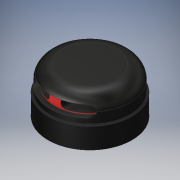
# Autodesk Inventor part: RPLidar A2
Saved by Autodesk Inventor 2018 (Build 220112000, 112)
## iProperties
Part Number: RPLidar A2
Material: Generisch
Document SubType Name: Modeling
Designer: Jochen Alt
Mass: 156.122 g
Surface Area: 240.31 cm^2
Volume: 156.122 cm^3
Density: 1 g/cm^3
Appearance: Glänzend - schwarz
Author: Jochen Alt
Autodesk Inventor part; units mm, degrees
ref_plane "YZ Plane" through (0, 0, 0) normal (1, 0, 0) x (0, 1, 0)
ref_plane "XZ Plane" through (0, 0, 0) normal (0, 1, 0) x (-1, 0, 0)
ref_plane "XY Plane" through (0, 0, 0) normal (0, 0, 1) x (1, 0, 0)
sketch "Skizze1" plane through (0, 0, 0) normal (0, 0, 1) x (1, 0, 0)
  circle A0 centre (0, 0) radius 37.85
  dimension "d0" = 75.7
  constraints: 1 centre point, 1 coincident
  measures "d0" diameter of A0
extrude "Extrusion1" add sketch "Skizze1" along normal blind 18.6
sketch "Skizze2" plane through (0, 0, 18.6) normal (0, 0, 1) x (1, 0, 0)
  circle A0 centre (0, 0) radius 37.85 projected
  circle A1 centre (0, 0) radius 27.5647
  constraints: 1 centre point, 1 coincident
extrude "Extrusion2" add sketch "Skizze2" along normal blind 0.8 contours A1
sketch "Skizze3" plane through (0, 0, 19.4) normal (0, 0, 1) x (1, 0, 0)
  circle A0 centre (0, 0) radius 27.5647 projected
  circle A1 centre (0, 0) radius 36.25
  dimension "d5" = 72.5
  constraints: 1 centre point, 1 coincident
  measures "d5" diameter of A1
extrude "Extrusion3" add sketch "Skizze3" along normal blind 21.4 contours A0 | A1
fillet "Rundung1" radius 12 1 edges at (-36.25, 0, 40.8)
sketch "Skizze4" plane through (0, 0, 0) normal (0, 1, 0) x (-1, 0, 0)
  line L0 (36.25, 28.8) -> (-36.25, 28.8) projected
  line L1 (23.5, 28.8) -> (-23.5, 28.8) construction
  line L2 (23.5, 33.8) -> (-23.5, 33.8)
  line L3 (-23.5, 23.8) -> (23.5, 23.8)
  arc A0 (23.5, 23.8) -> (23.5, 33.8) centre (23.5, 28.8) ccw
  arc A1 (-23.5, 33.8) -> (-23.5, 23.8) centre (-23.5, 28.8) ccw
  line L4 (0, -8.16) -> (0, 48.96) construction
  point P0 (0, 0)
  point P1 (0, 28.8)
  dimension "d9" = 10
  dimension "d10" = 47
  constraints: 8 end point, 4 point on circle, 4 tangent, 2 centre point, 2 point on line, 1 midpoint, 1 parallel, 1 other
  measures "d9" distance between parallel lines of L3 L2
  measures "d10" distance of L1.end L1.start
extrude "Extrusion4" cut sketch "Skizze4" against normal through all
sketch "Skizze5" plane through (0, 0, 19.4) normal (0, 0, -1) x (-1, 0, 0)
  circle A0 centre (0, 0) radius 27.5647 projected
  circle A1 centre (0, 0) radius 31.9541
  constraints: 1 centre point, 1 coincident
extrude "Extrusion5" add sketch "Skizze5" against normal blind 15 contours A0 | A1
sketch "Skizze6" plane through (0, 0, 0) normal (0, 1, 0) x (-1, 0, 0)
  line L0 (40.5995, 28.8) -> (-50.4498, 28.8) construction
  line L1 (36.25, 19.4) -> (-36.25, 19.4) construction
  line L2 (0, -8.16) -> (0, 48.96) construction
  line L3 (23, 28.8) -> (9, 28.8) construction
  line L4 (23, 32.8) -> (9, 32.8)
  line L5 (9, 24.8) -> (23, 24.8)
  arc A0 (23, 24.8) -> (23, 32.8) centre (23, 28.8) ccw
  arc A1 (9, 32.8) -> (9, 24.8) centre (9, 28.8) ccw
  line L6 (-9, 28.8) -> (-23, 28.8) construction
  line L7 (-9, 32.8) -> (-23, 32.8)
  line L8 (-23, 24.8) -> (-9, 24.8)
  arc A2 (-9, 24.8) -> (-9, 32.8) centre (-9, 28.8) ccw
  arc A3 (-23, 32.8) -> (-23, 24.8) centre (-23, 28.8) ccw
  point P0 (0, 0)
  point P1 (16, 28.8)
  point P2 (-16, 28.8)
  dimension "d15" = 9.4
  dimension "d16" = 14
  dimension "d17" = 10
  dimension "d20" = 8
  constraints: 18 end point, 8 point on circle, 8 tangent, 4 centre point, 4 point on line, 2 midpoint, 2 parallel, 1 collinear, 1 horizontal, 2 other
  measures "d15" distance between parallel lines of L1 L0
  measures "d16" distance of L6.end L6.start
  measures "d20" distance between parallel lines of L8 L7
extrude "Extrusion6" cut sketch "Skizze6" against normal through all
sketch "Skizze7" plane through (0, 0, 0) normal (0, 0, -1) x (-1, 0, 0)
  circle A0 centre (0, 0) radius 29.5 construction
  line L0 (20.8597, 20.8597) -> (-20.8597, 20.8597) construction
  line L1 (-20.8597, 20.8597) -> (-20.8597, -20.8597) construction
  line L2 (-20.8597, -20.8597) -> (20.8597, -20.8597) construction
  line L3 (20.8597, -20.8597) -> (20.8597, 20.8597) construction
  line L4 (20.8597, 20.8597) -> (-20.8597, -20.8597) construction
  line L5 (-20.8597, 20.8597) -> (20.8597, -20.8597) construction
  dimension "d21" = 59
  constraints: 12 end point, 5 coincident, 2 midpoint, 2 parallel, 2 perpendicular, 1 horizontal, 3 other
hole "Bohrung1" at (-20.8597, -20.8597, 0) at (20.8597, -20.8597, 0) at (20.8597, 20.8597, 0) at (-20.8597, 20.8597, 0) direction (0, 0, 1) diameter 3 depth 4 tip angle 118
